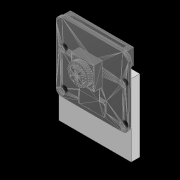
# Autodesk Inventor part: RPi_Camera_V2.1
Saved by Autodesk Inventor 2022 (Build 260153000, 153)
## iProperties
Created: 2021-09-27
Part Number: RPi_Camera_V2.1
Material: Genérico
Document SubType Name: Modeling
Designer: Julio R
Density: 1 g/cm^3
Appearance: Valor por defecto
Author: Julio R
Autodesk Inventor part; units mm, degrees
ref_plane "YZ Plane" through (0, 0, 0) normal (1, 0, 0) x (0, 1, 0)
ref_plane "XZ Plane" through (0, 0, 0) normal (0, 1, 0) x (-1, 0, 0)
ref_plane "Plano de trabajo1" through (10.95, 6.5, 0) normal (0, 0, -1) x (-1, 0, 0)
sketch "Boceto1" plane through (10.95, 6.5, 0) normal (0, 0, -1) x (-1, 0, 0)
  circle A0 centre (0.45, -4) radius 1.05 projected
  circle A1 centre (21.45, -4) radius 1.05 projected
  circle A2 centre (21.45, -16.58) radius 1.05 projected
  circle A3 centre (0.45, -16.58) radius 1.05 projected
  line L0 (-1.55, 3.5) -> (-1.55, -16.5) projected
  line L1 (0.45, -18.5) -> (21.45, -18.5) projected
  line L2 (23.45, -16.5) -> (23.45, 3.5) projected
  line L3 (-1.55, -2) -> (23.45, -2)
  line L4 (23.45, -2) -> (23.45, -27)
  line L5 (23.45, -27) -> (-1.55, -27)
  line L6 (-1.55, -27) -> (-1.55, -2)
  circle A4 centre (0.45, -4) radius 1.05
  circle A5 centre (21.45, -4) radius 1.05
  circle A6 centre (0.45, -16.58) radius 1.05
  circle A7 centre (21.45, -16.58) radius 1.05
  point P0 (10.95, -6.5)
  point P1 (0, 0)
  dimension "d1" = 2
  dimension "d3" = 25
  constraints: 8 end point, 4 centre point, 4 coincident, 4 concentric, 2 collinear, 2 parallel, 1 horizontal, 1 perpendicular, 1 point on line
  measures "d1" distance from line of L3 point (0, 0)
  measures "d3" distance between parallel lines of L3 L5
extrude "Extrusión1" add sketch "Boceto1" along normal blind 3
